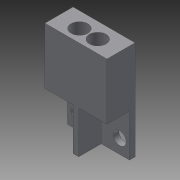
# Autodesk Inventor part: HVcup
Saved by Autodesk Inventor 2015 SP1 (Build 190203100, 203)
## iProperties
Created: 2015-10-07
Part Number: HVcup
Material: Generic
Document SubType Name: Modeling
Designer: I Rabey
Density: 1 g/cm^3
Appearance: Default
Author: I Rabey
Autodesk Inventor part; units mm, degrees
ref_plane "YZ Plane" through (0, 0, 0) normal (1, 0, 0) x (0, 1, 0)
ref_plane "XZ Plane" through (0, 0, 0) normal (0, 1, 0) x (-1, 0, 0)
ref_plane "XY Plane" through (0, 0, 0) normal (0, 0, 1) x (1, 0, 0)
sketch "Sketch1" plane through (0, 0, 0) normal (0, 0, 1) x (1, 0, 0)
  line L0 (-11, -17.5) -> (11, -17.5)
  line L1 (11, -17.5) -> (11, 17.5)
  line L2 (11, 17.5) -> (-11, 17.5)
  line L3 (-11, 17.5) -> (-11, -17.5)
  line L4 (-11, -17.5) -> (11, 17.5) construction
  line L5 (11, -17.5) -> (-11, 17.5) construction
  point P0 (0, 0)
  dimension "d0" = 22
  dimension "d1" = 35
  constraints: 12 end point, 2 midpoint, 2 parallel, 1 horizontal, 1 perpendicular
  measures "d0" distance of L2.end L1.end
  measures "d1" distance of L1.end L0.end
extrude "Extrusion1" add sketch "Sketch1" along normal blind 10
sketch "Sketch2" plane through (0, 0, 10) normal (0, 0, 1) x (1, 0, 0)
  line L0 (-11, -17.5) -> (19, -17.5)
  line L1 (19, -17.5) -> (19, -2.5)
  line L2 (19, -2.5) -> (-11, -2.5)
  line L3 (-11, -2.5) -> (-11, -17.5)
  point P0 (0, 0)
  dimension "d4" = 30
  dimension "d5" = 15
  constraints: 8 end point, 2 parallel, 1 horizontal, 1 perpendicular
  measures "d4" distance of L2.end L1.end
  measures "d5" distance of L1.end L0.end
extrude "Extrusion2" cut sketch "Sketch2" against normal blind 8
sketch "Sketch4" plane through (0, 0, 2) normal (0, 0, 1) x (1, 0, 0)
  circle A0 centre (-7.5, -12.5) radius 2.45
  circle A1 centre (7.5, -12.5) radius 2.45
  line L0 (11, -17.5) -> (-11, -17.5) projected
  point P0 (0, 0)
  dimension "d12" = 4.9
  dimension "d13" = 4.9
  dimension "d14" = 15
  dimension "d15" = 7.5
  dimension "d16" = 5
  dimension "d17" = 5
  constraints: 2 centre point
  measures "d12" diameter of A0
  measures "d13" diameter of A1
  measures "d14" distance of A1.centre A0.centre
  measures "d15" horizontal distance of point (0, 0) A0.centre
  measures "d16" distance from line of A0.centre L0
  measures "d17" distance from line of L0 A1.centre
hole "Hole1" at (-7.5, -12.5, 2) at (7.5, -12.5, 2) direction (0, 0, -1) diameter 4.6 end through all
sketch "Sketch5" plane through (-11, 17.5, 0) normal (0, 1, 0) x (1, 0, 0)
  circle A0 centre (7.75, -5.5) radius 2.95
  circle A1 centre (14.25, -5.5) radius 2.95
  line L0 (22, -10) -> (0, -10) projected
  point P0 (11, 0)
  dimension "d25" = 5.9
  dimension "d26" = 5.9
  dimension "d27" = 6.5
  dimension "d28" = 3.25
  dimension "d29" = 4.5
  dimension "d30" = 4.5
  constraints: 2 centre point
  measures "d25" diameter of A0
  measures "d26" diameter of A1
  measures "d27" distance of A1.centre A0.centre
  measures "d28" horizontal distance of point (11, 0) A0.centre
  measures "d29" distance from line of A0.centre L0
  measures "d30" distance from line of L0 A1.centre
extrude "Extrusion8" cut sketch "Sketch5" against normal blind 8
sketch "Sketch9" plane through (-11, -2.5, 2) normal (0, -1, 0) x (1, 0, 0)
  circle A0 centre (7.75, 3.5) radius 2.95 projected
  circle A1 centre (7.75, 3.5) radius 1.25
  point P0 (11, -2)
  dimension "d45" = 2.5
  constraints: 1 centre point, 1 coincident
  measures "d45" diameter of A1
extrude "Extrusion9" cut sketch "Sketch9" against normal up to next contours A1
sketch "Sketch13" plane through (-11, -2.5, 10) normal (0, -1, 0) x (1, 0, 0)
  circle A0 centre (14.25, -4.5) radius 2.95 projected
  circle A1 centre (14.25, -4.5) radius 1.25
  point P0 (11, -10)
  dimension "d58" = 2.5
  constraints: 1 centre point, 1 coincident
  measures "d58" diameter of A1
extrude "Extrusion13" cut sketch "Sketch13" against normal up to next contours A1
sketch "Sketch14" plane through (0, 0, 2) normal (0, 0, 1) x (1, 0, 0)
  line L0 (-11, -2.5) -> (11, -2.5) projected
  line L1 (-1, -2.5) -> (1, -2.5)
  line L2 (1, -2.5) -> (1, -17.5)
  line L3 (1, -17.5) -> (-1, -17.5)
  line L4 (-1, -17.5) -> (-1, -2.5)
  point P0 (0, 0)
  dimension "d61" = 2
  dimension "d62" = 15
  dimension "d63" = 1
  constraints: 8 end point, 2 parallel, 1 horizontal, 1 perpendicular, 1 point on line
  measures "d61" distance of L2.end L3.end
  measures "d62" distance of L1.end L2.end
  measures "d63" distance from line of L2 point (0, 0)
extrude "Extrusion14" add sketch "Sketch14" along normal blind 8
equation "\"d28\" = 0.5 * d27"
equation "\"d30\" = d29"
body "Solid1"
